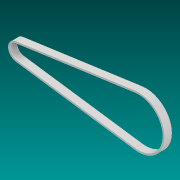
# Autodesk Inventor part: Tandriem20naar60T
Saved by Autodesk Inventor 2020.2 (Build 242310000, 310)
## iProperties
Created: 2020-05-14
Part Number: Tandriem20naar60T
Material: Generic
Document SubType Name: Modeling
Designer: Svend
Density: 1 g/cm^3
Appearance: Default
Author: Svend
Autodesk Inventor part; units mm, degrees
ref_plane "YZ Plane" through (0, 0, 0) normal (1, 0, 0) x (0, 1, 0)
ref_plane "XZ Plane" through (0, 0, 0) normal (0, 1, 0) x (-1, 0, 0)
ref_plane "XY Plane" through (0, 0, 0) normal (0, 0, 1) x (1, 0, 0)
sketch "Sketch1" plane through (0, 0, 0) normal (0, 0, 1) x (1, 0, 0)
  arc A0 (-0.8388, 5.9411) -> (-0.8388, -5.9411) centre (0, 0) ccw
  arc A1 (97.3474, -19.8036) -> (97.3474, 19.8036) centre (100.1434, 0) ccw
  line L0 (-0.8388, 5.9411) -> (97.3474, 19.8036)
  line L1 (-0.8388, -5.9411) -> (97.3474, -19.8036)
  line L2 (97.1657, 21.0908) -> (-1.0205, 7.2283)
  arc A2 (-1.0205, 7.2283) -> (-1.0205, -7.2283) centre (0, 0) ccw
  line L3 (-1.0205, -7.2283) -> (97.1657, -21.0908)
  arc A3 (97.1657, -21.0908) -> (97.1657, 21.0908) centre (100.1434, 0) ccw
  dimension "d0" = 12
  dimension "d1" = 40
  dimension "d2" = 99.16
  dimension "d3" = 1.3
  constraints: 8 end point, 8 point on circle, 4 centre point, 4 tangent, 1 coincident, 1 horizontal alignment, 3 other
  measures "d0" diameter of A0
  measures "d1" diameter of A1
  measures "d2" distance of L0.start L0.end
  measures "d3" distance between parallel lines of L0 L2
extrude "Extrusion1" add sketch "Sketch1" along normal mid plane 6
body "Solid1"
